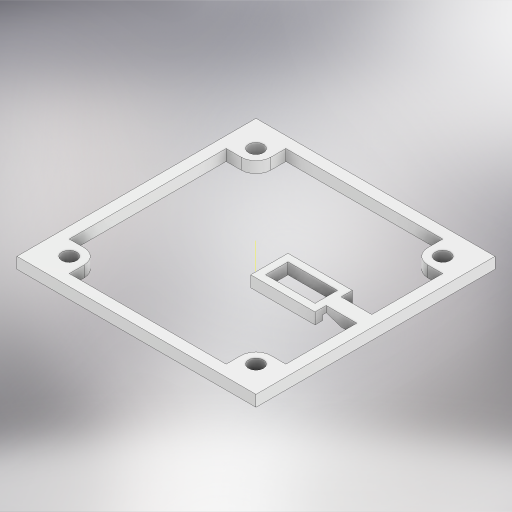
# Autodesk Inventor part: footprint
Saved by Autodesk Inventor 2024 (Build 280153000, 153)
## iProperties
Created: 2023-04-24
Part Number: footprint
Material: ABS Plastic
Document SubType Name: Modeling
Designer: byrne
Density: 1.06 g/cm^3
Appearance: Smooth - White
Author: byrne
Autodesk Inventor part; units mm, degrees
ref_plane "YZ Plane" through (0, 0, 0) normal (1, 0, 0) x (0, 1, 0)
ref_plane "XZ Plane" through (0, 0, 0) normal (0, 1, 0) x (-1, 0, 0)
ref_plane "XY Plane" through (0, 0, 0) normal (0, 0, 1) x (1, 0, 0)
sketch "Sketch3" plane through (0, 0, 0) normal (0, 1, 0) x (-1, 0, 0)
  line L0 (-50.8, 50.8) -> (50.8, 50.8)
  line L1 (50.8, 50.8) -> (50.8, -50.8)
  line L2 (50.8, -50.8) -> (-50.8, -50.8)
  line L3 (-50.8, -50.8) -> (-50.8, 50.8)
  line L4 (-50.8, 50.8) -> (50.8, -50.8) construction
  line L5 (50.8, 50.8) -> (-50.8, -50.8) construction
  line L6 (-46.0375, 46.0375) -> (46.0375, 46.0375)
  line L7 (46.0375, 46.0375) -> (46.0375, -46.0375)
  line L8 (46.0375, -46.0375) -> (-46.0375, -46.0375)
  line L9 (-46.0375, -46.0375) -> (-46.0375, 46.0375)
  point P0 (0, 0)
  dimension "d17" = 101.6
  dimension "d18" = 101.6
  dimension "d19" = 4.7625
  constraints: 20 end point, 4 parallel, 2 midpoint, 2 perpendicular, 1 horizontal, 3 other
  measures "d17" distance of L1.end L2.end
  measures "d18" distance of L0.end L1.end
  measures "d19" distance between parallel lines of L3 L9
extrude "Extrusion3" add sketch "Sketch3" along normal blind 4.7625
sketch "Sketch4" plane through (0, 0, 0) normal (0, -1, 0) x (1, 0, 0)
  line L0 (-50.8, 50.8) -> (50.8, 50.8)
  line L1 (50.8, 50.8) -> (50.8, -50.8)
  line L2 (50.8, -50.8) -> (-50.8, -50.8)
  line L3 (-50.8, -50.8) -> (-50.8, 50.8)
  line L4 (-50.8, 50.8) -> (50.8, -50.8) construction
  line L5 (50.8, 50.8) -> (-50.8, -50.8) construction
  line L6 (46.0375, -46.0375) -> (46.0375, 46.0375)
  line L7 (46.0375, 46.0375) -> (-46.0375, 46.0375)
  line L8 (-46.0375, 46.0375) -> (-46.0375, -46.0375)
  line L9 (-46.0375, -46.0375) -> (46.0375, -46.0375)
  circle A0 centre (39.6875, 39.6875) radius 3.175
  circle A1 centre (39.6875, 39.6875) radius 6.35
  line L10 (33.3375, 33.3375) -> (33.3159, 33.3375)
  line L11 (33.3375, 39.6875) -> (33.3375, 46.0375)
  line L12 (46.0375, 33.3375) -> (39.6875, 33.3375)
  point P0 (0, 0)
  dimension "d22" = 101.6
  dimension "d23" = 101.6
  dimension "d24" = 4.7625
  dimension "d25" = 6.35
  dimension "d26" = 3.175
  constraints: 26 end point, 5 tangent, 4 parallel, 3 horizontal, 3 point on line, 2 centre point, 2 midpoint, 2 perpendicular, 2 point on circle, 1 vertical, 3 other
  measures "d22" distance of L1.end L2.end
  measures "d23" distance of L0.end L1.end
  measures "d24" distance between parallel lines of L1 L6
  measures "d25" diameter of A0
  measures "d26" radial gap between concentric circles of A0 A1
extrude "Extrusion4" add sketch "Sketch4" against normal blind 4.7625 contours L12 A1 L6 | A1 L7 L6 | A1 | A1 L11 L7
pattern_circular "Circular Pattern1" count 4 over 360 about axis through (0, -10, 0) along (0, 1, 0) of "Extrusion4"
sketch "Sketch5" plane through (0, 0, 0) normal (0, -1, 0) x (1, 0, 0)
  circle A0 centre (25.4, 0) radius 1.75
  line L0 (9.35, 4.25) -> (29.35, 4.25)
  line L1 (29.35, 4.25) -> (29.35, -4.25)
  line L2 (29.35, -4.25) -> (9.35, -4.25)
  line L3 (9.35, -4.25) -> (9.35, 4.25)
  line L4 (-46.0375, -3.175) -> (46.0375, -3.175)
  line L5 (46.0375, -3.175) -> (46.0375, 3.175)
  line L6 (46.0375, 3.175) -> (-46.0375, 3.175)
  line L7 (-46.0375, 3.175) -> (-46.0375, -3.175)
  line L8 (-46.0375, -3.175) -> (46.0375, 3.175) construction
  line L9 (46.0375, -3.175) -> (-46.0375, 3.175) construction
  line L10 (29.85, -4.75) -> (29.85, 4.75)
  line L11 (29.85, 4.75) -> (8.85, 4.75)
  line L12 (8.85, 4.75) -> (8.85, -4.75)
  line L13 (8.85, -4.75) -> (29.85, -4.75)
  line L14 (33.025, -7.925) -> (33.025, 7.925)
  line L15 (33.025, 7.925) -> (5.675, 7.925)
  line L16 (5.675, 7.925) -> (5.675, -7.925)
  line L17 (5.675, -7.925) -> (33.025, -7.925)
  line L18 (46.0375, -33.3375) -> (46.0375, 33.3375) projected
  line L19 (50.8, 50.8) -> (50.8, -50.8) projected
  point P0 (0, 0)
  point P1 (29.35, 3.175)
  point P2 (29.35, -3.175)
  point P3 (9.35, -3.175)
  point P4 (9.35, 3.175)
  point P5 (33.025, 3.175)
  point P6 (5.675, 3.175)
  point P7 (5.675, -3.175)
  point P8 (33.025, -3.175)
  point P9 (46.0375, -46.0375)
  point P10 (46.0375, 46.0375)
  point P11 (29.35, 0)
  point P12 (46.0375, 0)
  point P13 (46.0375, 0)
  dimension "d33" = 3.5
  dimension "d34" = 20
  dimension "d35" = 92.075
  dimension "d38" = 0.5
  dimension "d39" = 3.175
  dimension "d72" = 25.4
  dimension "d73" = 3.95
  dimension "d74" = 8.5
  dimension "d75" = 6.35
  constraints: 36 end point, 8 parallel, 4 perpendicular, 3 midpoint, 2 horizontal, 2 horizontal alignment, 1 centre point, 1 coincident, 1 vertical, 6 other
  measures "d33" diameter of A0
  measures "d34" distance of L1.end L2.end
  measures "d35" distance of L5.end L6.end
  measures "d38" distance between parallel lines of L1 L10
  measures "d39" distance between parallel lines of L13 L17
  measures "d72" distance from line of L19 A0.centre
  measures "d73" distance from line of A0.centre L1
  measures "d74" distance of L0.end L1.end
  measures "d75" distance between parallel lines of L6 L4
extrude "Extrusion5" add sketch "Sketch5" against normal blind 4.7625 contours L12 L4 L16 L6 | L6 L16 L15 L14 L10 L11 L12 | L6 L14 L4 L10 | L12 L13 L10 L4 L14 L17 L16 | L6 L5 L4 L14
chamfer "Chamfer1" distance 9.525 distance2 3.175 1 edges at (29.85, 0, 0) measured on face at (30.35, 0, 0)
ref_plane "Work Plane2" through (-50.8, 0, 0) normal (0, 0, 1) x (1, 0, 0)
ref_plane "Work Plane3" through (0, 0, 50.8) normal (1, 0, 0) x (0, 0, -1)
body "Solid2"
